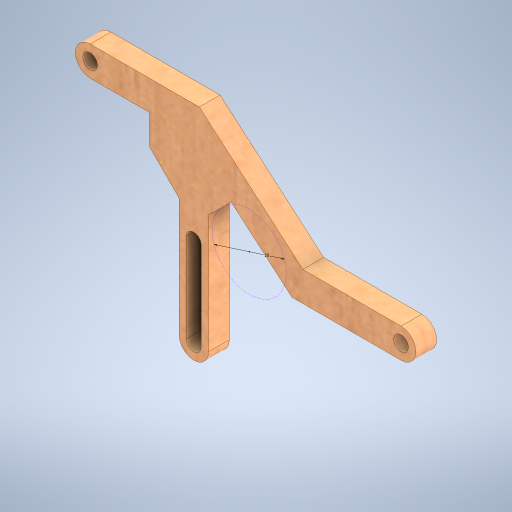
# Autodesk Inventor part: BrazoV2
Saved by Autodesk Inventor 2023.1 (Build 271208000, 208)
## iProperties
Created: 2022-10-30
Part Number: BrazoV2
Material: MDF Medium Density Fiberboard
Document SubType Name: Modeling
Designer: Daniel Peña
Density: 0.8 g/cm^3
Appearance: Cherry - Natural Low Gloss
Author: Daniel Peña
Autodesk Inventor part; units mm, degrees
ref_plane "YZ Plane" through (0, 0, 0) normal (1, 0, 0) x (0, 1, 0)
ref_plane "XZ Plane" through (0, 0, 0) normal (0, 1, 0) x (-1, 0, 0)
ref_plane "XY Plane" through (0, 0, 0) normal (0, 0, 1) x (1, 0, 0)
sketch "Sketch1" plane through (0, 0, 0) normal (0, 0, 1) x (1, 0, 0)
  line L0 (-24.0654, 17.5007) -> (10.9346, 17.5007) construction
  line L1 (45.9346, -12.4993) -> (80.9346, -12.4993) construction
  line L2 (10.9346, 17.5007) -> (45.9346, -12.4993) construction
  line L3 (-24.0654, 22.5007) -> (12.7842, 22.5007)
  line L4 (12.7842, 22.5007) -> (47.7842, -7.4993)
  line L5 (47.7842, -7.4993) -> (80.9346, -7.4993)
  line L6 (-24.0654, 12.5007) -> (-4.0654, 12.5007)
  line L7 (44.085, -17.4993) -> (80.9346, -17.4993)
  line L8 (10.9346, 17.5007) -> (10.9346, -47.4993) construction
  line L9 (15.9346, -7.4993) -> (15.9346, -47.4993)
  line L10 (22.4168, 1.0734) -> (44.085, -17.4993)
  arc A0 (-29.0654, 17.5007) -> (-24.0654, 12.5007) centre (-24.0654, 17.5007) ccw
  arc A1 (-24.0654, 22.5007) -> (-29.0654, 17.5007) centre (-24.0654, 17.5007) ccw
  arc A2 (85.9346, -12.4993) -> (80.9346, -7.4993) centre (80.9346, -12.4993) ccw
  arc A3 (80.9346, -17.4993) -> (85.9346, -12.4993) centre (80.9346, -12.4993) ccw
  arc A4 (10.9346, -52.4993) -> (15.9346, -47.4993) centre (10.9346, -47.4993) ccw
  arc A5 (5.9346, -47.4993) -> (10.9346, -52.4993) centre (10.9346, -47.4993) ccw
  line L11 (-4.0654, 12.5007) -> (-4.0654, 2.5007)
  line L12 (5.9346, -7.4993) -> (5.9346, -7.4993)
  line L13 (-4.0654, 2.5007) -> (5.9346, -7.4993)
  line L14 (15.9346, -7.4993) -> (23.5424, 0.1085)
  line L15 (5.9346, -47.4993) -> (5.9346, -7.4993)
  point P0 (0, 0)
  point P1 (-29.0654, 17.5007)
  point P2 (-4.0654, -7.4993)
  dimension "d0" = 35
  dimension "d4" = 35
  dimension "d5" = 35
  dimension "d6" = 30
  dimension "d7" = 5
  dimension "d8" = 5
  dimension "d10" = 5
  dimension "d11" = 5
  dimension "d13" = 65
  dimension "d14" = 5
  dimension "d15" = 5
  dimension "d16" = 5
  dimension "d34" = 5
  dimension "d35" = 5
  dimension "d36" = 5
  dimension "d37" = 5
  dimension "d41" = 20
  dimension "d43" = 10
  dimension "d44" = 10
  dimension "d47" = 135
  constraints: 32 end point, 12 point on circle, 6 centre point, 5 equal radius, 5 tangent, 3 coincident, 3 point on line, 3 vertical, 2 horizontal, 12 other
  measures "d0" distance of L0.start L0.end
  measures "d4" distance of L1.start L1.end
  measures "d5" horizontal distance of L1.start L0.end
  measures "d6" vertical distance of L1.start L0.end
  measures "d7" distance between parallel lines of L0 L3
  measures "d8" distance between parallel lines of L0 L6
  measures "d13" distance of L0.end L8.end
  measures "d14" distance between parallel lines of L9 L8
  measures "d16" radius of A0
  measures "d34" distance between parallel lines of L7 L1
  measures "d35" distance between parallel lines of L1 L5
  measures "d36" distance between parallel lines of L10 L2
  measures "d37" distance between parallel lines of L2 L4
  measures "d41" distance of L6.end point (-4.065, -7.499)
  measures "d43" distance of L11.end point (-4.065, -7.499)
  measures "d44" distance of L12.start point (-4.065, -7.499)
  measures "d47" angle of L9 L14
extrude "Cuerpo" add sketch "Sketch1" along normal blind 7
sketch "Sketch2" plane through (0, 0, 7) normal (0, 0, 1) x (1, 0, 0)
  arc A0 (-24.0654, 22.5007) -> (-24.0654, 12.5007) centre (-24.0654, 17.5007) ccw projected
  arc A1 (80.9346, -17.4993) -> (80.9346, -7.4993) centre (80.9346, -12.4993) ccw projected
  point P0 (0, 0)
  constraints: 2 coincident
hole "Hole1" at (-24.0654, 17.5007, 7) at (80.9346, -12.4993, 7) direction (0, 0, -1) diameter 5 end through all
sketch "Sketch3" plane through (0, 0, 7) normal (0, 0, 1) x (1, 0, 0)
  arc A0 (5.9346, -47.4993) -> (15.9346, -47.4993) centre (10.9346, -47.4993) ccw construction
  line L0 (10.9346, -47.4993) -> (10.9346, -17.4993) construction
  line L1 (10.9346, -14.9993) -> (10.9346, -14.9993)
  line L2 (13.4346, -17.4993) -> (13.4346, -47.4993)
  line L3 (10.9346, -49.9993) -> (10.9346, -49.9993)
  line L4 (8.4346, -47.4993) -> (8.4346, -17.4993)
  arc A1 (10.9346, -14.9993) -> (8.4346, -17.4993) centre (10.9346, -17.4993) ccw
  arc A2 (13.4346, -17.4993) -> (10.9346, -14.9993) centre (10.9346, -17.4993) ccw
  arc A3 (8.4346, -47.4993) -> (10.9346, -49.9993) centre (10.9346, -47.4993) ccw
  arc A4 (10.9346, -49.9993) -> (13.4346, -47.4993) centre (10.9346, -47.4993) ccw
  point P0 (0, 0)
  point P1 (10.9346, -14.9993)
  point P2 (10.9346, -49.9993)
  dimension "d26" = 30
  dimension "d28" = 2.5
  dimension "d29" = 2.5
  dimension "d30" = 2.5
  dimension "d31" = 2.5
  constraints: 10 end point, 8 point on circle, 8 tangent, 4 centre point, 3 equal radius, 2 parallel, 1 horizontal, 1 perpendicular, 1 vertical, 1 other
  measures "d26" distance of L0.start L0.end
  measures "d28" distance from line of L1 L0.end
  measures "d29" distance from line of L0.start L3
  measures "d30" distance between parallel lines of L4 L0
  measures "d31" radius of A1
extrude "Ranura" cut sketch "Sketch3" against normal blind 7
sketch "Sketch4" plane through (0, 0, 7) normal (0, 0, 1) x (1, 0, 0)
  circle A0 centre (29.6299, -11.3906) radius 12.5 construction
  point P0 (0, 0)
  dimension "d38" = 25
  constraints: 1 centre point
  measures "d38" diameter of A0
equation "\"d44\" = d43"
body "Solid1"
